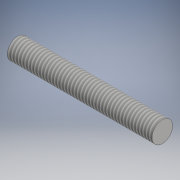
# Autodesk Inventor part: Forefingers Rod4
Saved by Autodesk Inventor 2017 (Build 210142000, 142)
## iProperties
Created: 2017-11-01
Part Number: Forefingers Rod4
Material: Generic
Document SubType Name: Modeling
Designer: julie
Density: 1 g/cm^3
Appearance: Default
Author: julie
Autodesk Inventor part; units mm, degrees
ref_plane "YZ Plane" through (0, 0, 0) normal (1, 0, 0) x (0, 1, 0)
ref_plane "XZ Plane" through (0, 0, 0) normal (0, 1, 0) x (-1, 0, 0)
ref_plane "XY Plane" through (0, 0, 0) normal (0, 0, 1) x (1, 0, 0)
sketch "Sketch1" plane through (0, 0, 0) normal (1, 0, 0) x (0, 1, 0)
  circle A0 centre (0, 0) radius 2.5
  dimension "d0" = 5
  constraints: 1 centre point, 1 coincident
  measures "d0" diameter of A0
extrude "Extrusion1" add sketch "Sketch1" along normal blind 35
thread "Thread1" size "3/8-32 UNEF" class "2A" standard "ANSI Unified Screw Threads" full length
body "Solid1"
